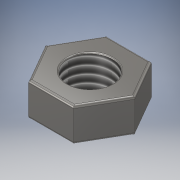
# Autodesk Inventor part: M4 Nut
Saved by Autodesk Inventor 2018 (Build 220112000, 112)
## iProperties
Created: 2018-05-02
Part Number: M4 Nut
Material: Stainless Steel
Document SubType Name: Modeling
Designer: Ajith Thomas
Mass: 0.713129 g
Surface Area: 1.64911 cm^2
Volume: 0.0891411 cm^3
Density: 8 g/cm^3
Appearance: Semi-Polished
Author: Ajith Thomas
Autodesk Inventor part; units mm, degrees
ref_plane "YZ Plane" through (0, 0, 0) normal (1, 0, 0) x (0, 1, 0)
ref_plane "XZ Plane" through (0, 0, 0) normal (0, 1, 0) x (-1, 0, 0)
ref_plane "XY Plane" through (0, 0, 0) normal (0, 0, 1) x (1, 0, 0)
sketch "Sketch1" plane through (0, 0, 0) normal (0, 1, 0) x (-1, 0, 0)
  circle A0 centre (0, 0) radius 3.5 construction
  line L0 (-2.0207, -3.5) -> (-4.0415, 0)
  line L1 (-4.0415, 0) -> (-2.0207, 3.5)
  line L2 (-2.0207, 3.5) -> (2.0207, 3.5)
  line L3 (2.0207, 3.5) -> (4.0415, 0)
  line L4 (4.0415, 0) -> (2.0207, -3.5)
  line L5 (2.0207, -3.5) -> (-2.0207, -3.5)
  point P0 (0, -3.5)
  dimension "d0" = 7
  constraints: 12 end point, 2 coincident, 1 midpoint, 1 vertical alignment, 15 other
extrude "Extrusion1" add sketch "Sketch1" along normal mid plane 3
sketch "Sketch2" plane through (0, 1.5, 0) normal (0, 1, 0) x (1, 0, 0)
  circle A0 centre (0, 0) radius 2
  dimension "d3" = 4
  constraints: 1 centre point, 1 coincident
  measures "d3" diameter of A0
extrude "Extrusion2" cut sketch "Sketch2" against normal blind 3
fillet "Fillet1" radius 0.2 12 edges at (-3.0311, 1.5, 1.75) (0, 1.5, 3.5) (3.0311, 1.5, 1.75) (3.0311, 1.5, -1.75) (0, 1.5, -3.5) (-3.0311, 1.5, -1.75) (0, -1.5, 3.5) (-3.0311, -1.5, 1.75) (-3.0311, -1.5, -1.75) (0, -1.5, -3.5) (3.0311, -1.5, -1.75) (3.0311, -1.5, 1.75)
fillet "Fillet2" radius 0.1 2 edges at (-2, 1.5, 0) (-2, -1.5, 0)
thread "Thread1" size "M4x0.7" class "6H" standard "ANSI Metric M Profile" full length
body "Solid1"
